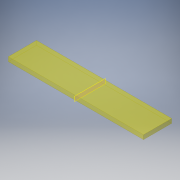
# Autodesk Inventor part: rearBox
Saved by Autodesk Inventor 2016 SP1 (Build 200210100, 210)
## iProperties
Created: 2016-01-20
Part Number: rearBox
Material: Wood (Walnut)
Document SubType Name: Modeling
Designer: steele
Density: 0.55 g/cm^3
Appearance: Clear - Yellow
Author: steele
Autodesk Inventor part; units mm, degrees
ref_plane "XZ Plane" through (0, 0, 0) normal (0, 1, 0) x (-1, 0, 0)
ref_plane "XY Plane" through (0, 0, 0) normal (0, 0, 1) x (1, 0, 0)
sketch "Sketch1" plane through (0, 0, 0) normal (0, 1, 0) x (-1, 0, 0)
  line L0 (304.8, 63.5) -> (-304.8, 63.5)
  line L1 (-304.8, 63.5) -> (-304.8, -63.5)
  line L2 (-304.8, -63.5) -> (304.8, -63.5)
  line L3 (304.8, -63.5) -> (304.8, 63.5)
  line L4 (304.8, 63.5) -> (-304.8, -63.5) construction
  line L5 (-304.8, 63.5) -> (304.8, -63.5) construction
  point P0 (0, 0)
  dimension "d0" = 127
  dimension "d1" = 609.6
  constraints: 12 end point, 2 midpoint, 2 parallel, 1 horizontal, 1 perpendicular
  measures "d0" distance of L0.end L1.end
  measures "d1" distance of L0.start L0.end
extrude "Extrusion1" add sketch "Sketch1" along normal blind 19.05
equation "\"d0\" = rearBoxLegth"
equation "\"d1\" = rearBoxWidth"
equation "\"d2\" = rearBoxThickness"
equation "\"rearBoxWidth\" = 609.6"
equation "\"rearBoxLegth\" = 127"
equation "\"rearBoxThickness\" = 19.05"
body "Solid1"
